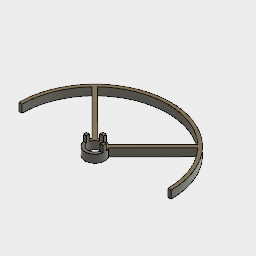
四轴护罩部件01 (Autodesk Fusion 360 design; units mm, degrees)
Autodesk Fusion 360 part; units mm, degrees
note: some values were not read from the file. Chosen so that the rebuilt part matches the saved one: which face or edge a step refers to.
sketch "草图1" plane through (0, 0, 0) normal (0, 1, 0) x (1, 0, 0)
  circle A0 centre (0, 0) radius 4.4
  circle A1 centre (0, 0) radius 6.25
  line L0 (-5.2189, 3.4388) -> (-3.4537, 5.2091)
  line L1 (-3.4537, 5.2091) -> (-32.4862, 34.1592)
  line L2 (-32.4862, 34.1592) -> (-34.2515, 32.389)
  line L3 (-34.2515, 32.389) -> (-5.2189, 3.4388)
  line L4 (5.2067, 3.4573) -> (3.4351, 5.2213)
  line L5 (3.4351, 5.2213) -> (32.3647, 34.2744)
  line L6 (32.3647, 34.2744) -> (34.1362, 32.5104)
  line L7 (34.1362, 32.5104) -> (5.2067, 3.4573)
  arc A2 (45.8929, 0.0909) -> (-45.893, -0.0459) centre (0, 0) ccw
  arc A3 (47.9999, 0.1111) -> (-48, -0.0423) centre (0, 0) ccw
  line L8 (-48, -0.0423) -> (-45.893, -0.0459)
  line L9 (45.8929, 0.0909) -> (47.9999, 0.1111)
  dimension "d1" = 8.8
  dimension "d2" = 12.5
  dimension "d3" = 41
  dimension "d4" = 41
  dimension "d5" = 45.893
  dimension "d11" = 2.5
  dimension "d12" = 2.5
  dimension "d13" = 48
  measures "d1" diameter of A0
  measures "d2" diameter of A1
  measures "d3" distance of L0.start L2.end
  measures "d4" distance of L4.start L6.end
  measures "d5" radius of A2
  measures "d11" distance of L1.end L2.end
  measures "d12" distance of L5.end L6.end
  measures "d13" radius of A3
extrude "拉伸5" add sketch "草图1" along normal blind 5 contours A1 L0 L4 | A1 L4 | A1 L5 L7 A2 | A1 L1 L3 A2 | A1 L0 | L5 L6 L7 A2 | L1 L2 L3 L5 L6 L7 A2 A3 L8 L9 | L1 L2 L3 A2
sketch "草图2" plane through (0, 5, 0) normal (0, 1, 0) x (-1, 0, 0)
  arc A0 (-3.4351, -5.2213) -> (3.4537, -5.2091) centre (0, 0) ccw
  line L0 (3.4537, -5.2091) -> (31.6027, -33.2782)
  arc A1 (-31.4843, -33.3903) -> (31.6027, -33.2782) centre (0, 0) ccw
  line L1 (-31.4843, -33.3903) -> (-3.4351, -5.2213)
  circle A2 centre (0, 0) radius 4.4
  arc A3 (-45.8929, -0.0909) -> (-33.2558, -31.6263) centre (0, 0) ccw
  line L2 (-45.8929, -0.0909) -> (-47.9999, -0.1111)
  arc A4 (-47.9999, -0.1111) -> (48, 0.0423) centre (0, 0) ccw
  line L3 (48, 0.0423) -> (45.893, 0.0459)
  arc A5 (33.3679, -31.5079) -> (45.893, 0.0459) centre (0, 0) ccw
  line L4 (33.3679, -31.5079) -> (5.2189, -3.4388)
  arc A6 (5.2189, -3.4388) -> (-5.2067, -3.4573) centre (0, 0) ccw
  line L5 (-5.2067, -3.4573) -> (-33.2558, -31.6263)
  line L6 (-1.2389, -3.7783) -> (1.2611, -3.7783)
  line L7 (1.2611, -3.7783) -> (1.2611, -6.4499)
  line L8 (1.2611, -6.4499) -> (-1.2389, -6.4499)
  line L9 (-1.2389, -6.4499) -> (-1.2389, -3.7783)
  line L10 (-1.2389, -3.7783) -> (1.2611, -6.4499) construction
  line L11 (1.2611, -3.7783) -> (-1.2389, -6.4499) construction
  line L12 (3.5, 1) -> (6.9, 1)
  line L13 (6.9, 1) -> (6.9, -1)
  line L14 (6.9, -1) -> (3.5, -1)
  line L15 (3.5, -1) -> (3.5, 1)
  line L16 (3.5, 1) -> (6.9, -1) construction
  line L17 (6.9, 1) -> (3.5, -1) construction
  line L18 (-7.2149, 1) -> (-3.7851, 1)
  line L19 (-3.7851, 1) -> (-3.7851, -1)
  line L20 (-3.7851, -1) -> (-7.2149, -1)
  line L21 (-7.2149, -1) -> (-7.2149, 1)
  line L22 (-7.2149, 1) -> (-3.7851, -1) construction
  line L23 (-3.7851, 1) -> (-7.2149, -1) construction
  point P0 (0.0111, -5.1141)
  point P1 (5.2, 0)
  point P2 (-5.5, 0)
  dimension "d23" = 2.5
  dimension "d26" = 2
  dimension "d27" = 2
  measures "d23" distance of L7.end L8.end
  measures "d26" distance of L12.end L13.end
  measures "d27" distance of L18.end L19.end
sketch "草图7" plane through (0, 5, 0) normal (0, 1, 0) x (-1, 0, 0)
extrude "拉伸11" add sketch "草图2" along normal blind 3 contours A0 A2 L7 L9 | A2 A6 L18 L20 | A2 A6 L12 L14
extrude "拉伸12" add sketch "草图2" along normal blind 1 contours A0 L0 A1 L1 A2 A3 L2 A4 L3 A5 L4 A6 L5 L7 L9 L14 L20 | A2 A6 L12 L18
extrude "拉伸13" add 3 faces at (-0.0114, 8, -5.6239) (-5.6274, 8, 0) (5.6274, 8, 0) along direction (0, 1, 0) blind 2
extrude "拉伸14" cut 1 faces at (-0.0114, 10, -5.6239) along direction (0, -1, 0) blind 4
extrude "拉伸15" cut 1 faces at (-5.6274, 10, 0) along direction (0, -1, 0) blind 4
extrude "拉伸16" cut 1 faces at (5.6274, 10, 0) along direction (0, -1, 0) blind 4
extrude "拉伸17" add sketch "草图1" along normal blind 6 contours A0
extrude "拉伸18" cut 1 faces at (0.4169, 6, -1.5484) along direction (0, -1, 0) blind 1
extrude "拉伸19" cut sketch "草图1" along normal blind 5 contours A0
extrude "拉伸20" add sketch "草图2" along normal blind 4 contours A0 A2 L7 L9 | A2 A6 L18 L20 | A2 A6 L12 L14
sketch "草图15" plane through (0, 5, 0) normal (0, 1, 0) x (-1, 0, 0)
  line L0 (-4.2849, -1) -> (-6.1695, -1)
  arc A0 (-6.1695, -1) -> (-5.2067, -3.4573) centre (0, 0) ccw
  line L1 (-5.2067, -3.4573) -> (-33.2558, -31.6263)
  arc A1 (-45.8929, -0.0909) -> (-33.2558, -31.6263) centre (0, 0) ccw
  line L2 (-45.8929, -0.0909) -> (-47.9999, -0.1111)
  arc A2 (-47.9999, -0.1111) -> (48, 0.0423) centre (0, 0) ccw
  line L3 (48, 0.0423) -> (45.893, 0.0459)
  arc A3 (33.3679, -31.5079) -> (45.893, 0.0459) centre (0, 0) ccw
  line L4 (33.3679, -31.5079) -> (5.2189, -3.4388)
  arc A4 (5.2189, -3.4388) -> (6.1695, -1) centre (0, 0) ccw
  line L5 (6.1695, -1) -> (4.2849, -1)
  arc A5 (1.2611, -4.2154) -> (4.2849, -1) centre (0, 0) ccw
  line L6 (1.2611, -4.2154) -> (1.2611, -6.1214)
  arc A6 (1.2611, -6.1214) -> (3.4537, -5.2091) centre (0, 0) ccw
  line L7 (3.4537, -5.2091) -> (31.6027, -33.2782)
  arc A7 (-31.4843, -33.3903) -> (31.6027, -33.2782) centre (0, 0) ccw
  line L8 (-31.4843, -33.3903) -> (-3.4351, -5.2213)
  arc A8 (-3.4351, -5.2213) -> (-1.2389, -6.126) centre (0, 0) ccw
  line L9 (-1.2389, -6.126) -> (-1.2389, -4.222)
  arc A9 (-4.2849, -1) -> (-1.2389, -4.222) centre (0, 0) ccw
extrude "拉伸10" [suppressed]
extrude "拉伸6" [suppressed]
extrude "拉伸7" [suppressed]
extrude "拉伸8" [suppressed]
sketch "草图4" plane through (0, 3, 0.0923) normal (0, 1, 0) x (-1, 0, 0)
sketch "草图5" plane through (0, 6, 0) normal (0, 1, 0) x (-1, 0, 0)
  line L0 (4.1307, -1) -> (6.1695, -1)
  arc A0 (6.1695, -1) -> (6.1695, 1) centre (0, 0) ccw
  line L1 (6.1695, 1) -> (4.1307, 1)
  arc A1 (4.1307, -1) -> (4.1307, 1) centre (0, 0) ccw
  circle A2 centre (0, 0) radius 4.5
  dimension "d32" = 9
  measures "d32" diameter of A2
extrude "拉伸9" [suppressed]
extrude "拉伸1" [suppressed]
extrude "拉伸2" [suppressed]
extrude "拉伸3" [suppressed]
extrude "拉伸4" [suppressed]
